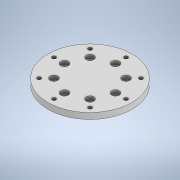
# Autodesk Inventor part: Adapter_bearing_link
Saved by Autodesk Inventor 2021 (Build 250183000, 183)
## iProperties
Created: 2020-05-19
Part Number: Adapter_bearing_link
Material: Generic
Document SubType Name: Modeling
Designer: Motius
Density: 1 g/cm^3
Appearance: Default
Author: Motius
Autodesk Inventor part; units mm, degrees
ref_plane "XZ Plane" through (0, 0, 0) normal (0, 1, 0) x (-1, 0, 0)
ref_plane "XY Plane" through (0, 0, 0) normal (0, 0, 1) x (1, 0, 0)
sketch "Sketch1" plane through (0, 0, 0) normal (0, 0, 1) x (1, 0, 0)
  line L0 (0, 5.9) -> (0, -17.9) construction
  line L1 (-7, 0) -> (42, 0) construction
  line L2 (0, -14.5) -> (0, 2.5)
  line L3 (0, -14.5) -> (6, -14.5)
  line L4 (6, -14.5) -> (6, -3.5)
  line L5 (7, -2.5) -> (35, -2.5)
  line L6 (35, -2.5) -> (35, 2.5)
  line L7 (35, 2.5) -> (0, 2.5)
  arc A0 (7, -2.5) -> (6, -3.5) centre (7, -3.5) ccw
  point P0 (0, 0)
  point P1 (6, -2.5)
  dimension "d0" = 6
  dimension "d2" = 5
  dimension "d3" = 12
  dimension "d4" = 1
  dimension "d12" = 35
  constraints: 12 end point, 4 perpendicular, 3 point on line, 2 point on circle, 2 tangent, 1 centre point, 1 vertical, 1 other
  measures "d0" distance of L2.start L3.end
  measures "d2" distance of L5.end L6.end
  measures "d3" distance between parallel lines of L5 L3
  measures "d4" radius of A0
  measures "d12" distance between parallel lines of L6 L0
revolve "Revolution1" add sketch "Sketch1" angle 360 about axis through (0, 0, 0) along (0, -1, 0)
sketch "Sketch2" plane through (0, 2.5, 0) normal (0, -1, 0) x (1, 0, 0)
  circle A0 centre (0, 0) radius 35 construction
  circle A1 centre (0, 0) radius 7 construction
  circle A2 centre (0, 0) radius 6 construction
  line L0 (-49, 0) -> (49, 0) construction
  line L1 (0, 49) -> (0, -49) construction
  circle A3 centre (0, 0) radius 6 construction
  circle A4 centre (0, 0) radius 21.25 construction
  circle A5 centre (0, 0) radius 30 construction
  point P0 (0, 30)
  point P1 (0, 21.25)
  point P2 (-21.2132, 21.2132)
  point P3 (-15.026, 15.026)
  point P4 (-30, 0)
  point P5 (-21.25, 0)
  point P6 (-21.2132, -21.2132)
  point P7 (-15.026, -15.026)
  point P8 (0, -30)
  point P9 (0, -21.25)
  point P10 (21.2132, -21.2132)
  point P11 (15.026, -15.026)
  point P12 (30, 0)
  point P13 (21.25, 0)
  point P14 (21.2132, 21.2132)
  point P15 (15.026, 15.026)
  dimension "d6" = 42.5
  dimension "d7" = 60
  dimension "d10" = 360
  constraints: 2 coincident, 2 point on line, 2 vertical alignment, 21 other
hole "Hole1" at (-15.026, 2.5, 15.026) at (0, 2.5, 21.25) at (15.026, 2.5, 15.026) at (21.25, 2.5, 0) at (15.026, 2.5, -15.026) at (0, 2.5, -21.25) at (-15.026, 2.5, -15.026) at (-21.25, 2.5, 0) direction (0, -1, 0) diameter 3.4 end through all counterbore diameter 6.5 counterbore depth 3 clearance for "Socket Head Cap Screw" size "M3" standard "Ansi Metric M Profile"
hole "Hole2" at (0, 2.5, 30) at (-21.2132, 2.5, 21.2132) at (-30, 2.5, 0) at (-21.2132, 2.5, -21.2132) at (0, 2.5, -30) at (21.2132, 2.5, -21.2132) at (30, 2.5, 0) at (21.2132, 2.5, 21.2132) direction (0, -1, 0) diameter 3.242 end through all thread size "M4x0.7" class "6H" standard "ANSI Metric M Profile"
ref_plane "Work Plane1" through (-6, -9, 0) normal (1, 0, 0) x (0, 1, 0)
sketch "Sketch3" plane through (-6, -9, 0) normal (1, 0, 0) x (0, 1, 0)
  line L0 (-8.9, 0) -> (14.9, 0) construction
  line L1 (-2.5, -2) -> (2.5, -2)
  line L2 (2.5, 2) -> (-2.5, 2)
  arc A0 (-2.5, 2) -> (-2.5, -2) centre (-2.5, 0) ccw
  arc A1 (2.5, -2) -> (2.5, 2) centre (2.5, 0) ccw
  line L3 (5.5, 6) -> (5.5, -6) construction
  line L4 (-5.5, 6) -> (-5.5, -6) construction
  line L5 (5.5, 6) -> (-5.5, 6) construction
  line L6 (0, 6) -> (0, -7.95) construction
  point P0 (9, 0)
  dimension "d27" = 4
  dimension "d29" = 5
  constraints: 6 end point, 4 point on circle, 4 tangent, 2 centre point, 1 horizontal, 1 midpoint, 1 parallel, 1 symmetric about line, 1 vertical, 1 other
  measures "d27" distance between parallel lines of L2 L1
  measures "d29" distance of A1.centre A0.centre
extrude "Extrusion1" cut sketch "Sketch3" along normal blind 2
chamfer "Chamfer1" distance 0.5 angle 45 1 edges at (-6, -14.5, 0)
body "Solid1"
